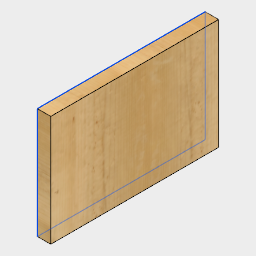
Short Side (Autodesk Fusion 360 design; units mm, degrees)
Autodesk Fusion 360 part; units mm, degrees
sketch "sketch 259" plane through (0, 0, 0) normal (1, 0, 0) x (0, 0, -1)
  line L0 (0, 209.55) -> (0, 0)
  line L1 (0, 0) -> (317.5, 0)
  line L2 (317.5, 0) -> (317.5, 209.55)
  line L3 (317.5, 209.55) -> (0, 209.55)
extrude "Extrude1" add sketch "sketch 259" along normal blind 25.4
